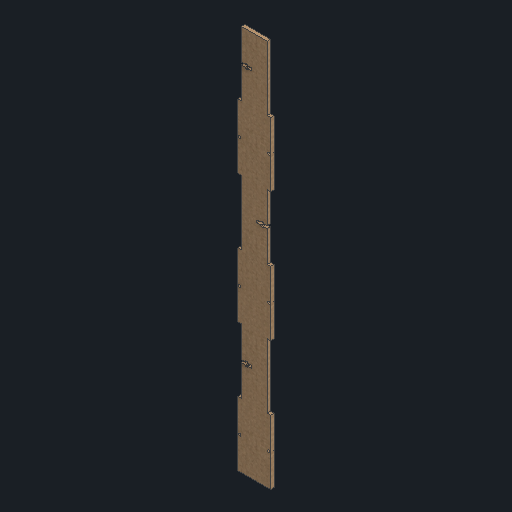
# Autodesk Inventor part: Cableduct_Cover
Saved by Autodesk Inventor 2024.1 (Build 281209000, 209)
## iProperties
Created: 2023-08-04
Part Number: Cableduct_Cover
Material: MDF Medium Density Fiberboard
Document SubType Name: Modeling
Designer: jaege
Density: 0.8 g/cm^3
Appearance: Cardboard - Corrugated
Author: jaege
Autodesk Inventor part; units mm, degrees
ref_plane "YZ Plane" through (0, 0, 0) normal (1, 0, 0) x (0, 1, 0)
ref_plane "XZ Plane" through (0, 0, 0) normal (0, 1, 0) x (-1, 0, 0)
ref_plane "XY Plane" through (0, 0, 0) normal (0, 0, 1) x (1, 0, 0)
sketch "Sketch1" plane through (0, 0, 0) normal (0, 0, 1) x (1, 0, 0)
  line L0 (75.5009, -337.6029) -> (75.5009, -262.6029) projected
  line L1 (71.5009, -262.6029) -> (75.5009, -262.6029) projected
  line L2 (71.5009, -337.6029) -> (71.5009, -262.6029) projected
  line L3 (71.5009, -337.6029) -> (75.5009, -337.6029) projected
  line L4 (75.5009, -187.6029) -> (75.5009, -112.6029) projected
  line L5 (71.5009, -112.6029) -> (75.5009, -112.6029) projected
  line L6 (71.5009, -187.6029) -> (71.5009, -112.6029) projected
  line L7 (71.5009, -187.6029) -> (75.5009, -187.6029) projected
  line L8 (75.5009, -37.6029) -> (75.5009, 37.3971) projected
  line L9 (71.5009, 37.3971) -> (75.5009, 37.3971) projected
  line L10 (71.5009, -37.6029) -> (71.5009, 37.3971) projected
  line L11 (71.5009, -37.6029) -> (75.5009, -37.6029) projected
  line L12 (75.5009, 37.3971) -> (105.5009, 37.3971)
  line L13 (105.5009, 37.3971) -> (105.5009, -412.6029)
  line L14 (105.5009, -412.6029) -> (75.5009, -412.6029)
  line L15 (75.5009, -412.6029) -> (75.5009, 37.3971)
  line L16 (71.5009, -412.6029) -> (279.5009, -412.6029) construction
  line L17 (90.5009, -412.6029) -> (90.5009, 37.3971) construction
  line L18 (105.5009, -337.6029) -> (105.5009, -262.6029)
  line L19 (109.5009, -262.6029) -> (105.5009, -262.6029)
  line L20 (109.5009, -337.6029) -> (109.5009, -262.6029)
  line L21 (109.5009, -337.6029) -> (105.5009, -337.6029)
  line L22 (105.5009, -187.6029) -> (105.5009, -112.6029)
  line L23 (109.5009, -112.6029) -> (105.5009, -112.6029)
  line L24 (109.5009, -187.6029) -> (109.5009, -112.6029)
  line L25 (109.5009, -187.6029) -> (105.5009, -187.6029)
  line L26 (105.5009, -37.6029) -> (105.5009, 37.3971)
  line L27 (109.5009, 37.3971) -> (105.5009, 37.3971)
  line L28 (109.5009, -37.6029) -> (109.5009, 37.3971)
  line L29 (109.5009, -37.6029) -> (105.5009, -37.6029)
  line L30 (71.5009, -37.6029) -> (71.5009, -112.6029)
  line L31 (71.5009, -187.6029) -> (71.5009, -262.6029)
  line L32 (71.5009, -337.6029) -> (71.5009, -412.6029)
  line L33 (75.5009, -412.6029) -> (71.5009, -412.6029)
  line L34 (109.5009, -337.6029) -> (109.5009, -412.6029)
  line L35 (109.5009, -412.6029) -> (105.5009, -412.6029)
  line L36 (109.5009, -262.6029) -> (109.5009, -187.6029)
  line L37 (109.5009, -112.6029) -> (109.5009, -37.6029)
  line L38 (71.5009, -37.6029) -> (75.5009, -112.6029) construction
  circle A0 centre (73.5009, -75.1029) radius 1.5
  circle A1 centre (73.5009, -225.1029) radius 1.5
  circle A2 centre (73.5009, -375.1029) radius 1.5
  circle A3 centre (107.5009, -75.1029) radius 1.5
  circle A4 centre (107.5009, -225.1029) radius 1.5
  circle A5 centre (107.5009, -375.1029) radius 1.5
  line L39 (75.5009, -1.6029) -> (87.5009, -1.6029)
  line L40 (87.5009, -1.6029) -> (87.5009, 1.3971)
  line L41 (87.5009, 1.3971) -> (75.5009, 1.3971)
  line L42 (75.5009, 1.3971) -> (75.5009, -1.6029)
  line L43 (82.7009, 2.5971) -> (80.3009, 2.5971)
  line L44 (80.3009, 2.5971) -> (80.3009, -2.8029)
  line L45 (80.3009, -2.8029) -> (82.7009, -2.8029)
  line L46 (82.7009, -2.8029) -> (82.7009, 2.5971)
  line L47 (93.5009, -151.6029) -> (105.5009, -151.6029)
  line L48 (105.5009, -151.6029) -> (105.5009, -148.6029)
  line L49 (105.5009, -148.6029) -> (93.5009, -148.6029)
  line L50 (93.5009, -148.6029) -> (93.5009, -151.6029)
  line L51 (100.7009, -147.4029) -> (98.3009, -147.4029)
  line L52 (98.3009, -147.4029) -> (98.3009, -152.8029)
  line L53 (98.3009, -152.8029) -> (100.7009, -152.8029)
  line L54 (100.7009, -152.8029) -> (100.7009, -147.4029)
  line L55 (75.5009, -301.6029) -> (87.5009, -301.6029)
  line L56 (87.5009, -301.6029) -> (87.5009, -298.6029)
  line L57 (87.5009, -298.6029) -> (75.5009, -298.6029)
  line L58 (75.5009, -298.6029) -> (75.5009, -301.6029)
  line L59 (82.7009, -297.4029) -> (80.3009, -297.4029)
  line L60 (80.3009, -297.4029) -> (80.3009, -302.8029)
  line L61 (80.3009, -302.8029) -> (82.7009, -302.8029)
  line L62 (82.7009, -302.8029) -> (82.7009, -297.4029)
  point P0 (87.5009, -0.1029)
  point P1 (71.5009, -0.1029)
  point P2 (82.7009, -0.1029)
  point P3 (81.5009, 2.5971)
  point P4 (81.5009, -1.6029)
  point P5 (105.5009, -150.1029)
  point P6 (100.7009, -150.1029)
  point P7 (99.5009, -147.4029)
  point P8 (99.5009, -151.6029)
  point P9 (87.5009, -300.1029)
  point P10 (82.7009, -300.1029)
  point P11 (81.5009, -297.4029)
  point P12 (81.5009, -301.6029)
  point P13 (109.5009, -150.1029)
  point P14 (71.5009, -300.1029)
  point P15 (80.3009, 1.3971)
  point P16 (82.7009, 1.3971)
  point P17 (82.7009, -1.6029)
  point P18 (80.3009, -1.6029)
  point P19 (80.3009, -298.6029)
  point P20 (82.7009, -298.6029)
  point P21 (82.7009, -301.6029)
  point P22 (80.3009, -301.6029)
  point P23 (100.7009, -151.6029)
  point P24 (98.3009, -151.6029)
  point P25 (98.3009, -148.6029)
  point P26 (100.7009, -148.6029)
  dimension "d3" = 30
  dimension "d4" = 3
  dimension "d7" = 150
  dimension "d10" = 34
  dimension "d13" = 3
  dimension "d14" = 12
  dimension "d15" = 5.4
  dimension "d16" = 2.4
  dimension "d17" = 3
  dimension "d18" = 12
  dimension "d19" = 5.4
  dimension "d20" = 2.4
  dimension "d21" = 3
  dimension "d22" = 12
  dimension "d23" = 5.4
  dimension "d24" = 2.4
  constraints: 100 end point, 18 equal length, 18 midpoint, 11 symmetric about line, 10 perpendicular, 8 horizontal, 7 horizontal alignment, 6 centre point, 5 vertical alignment, 3 point on line, 2 vertical, 10 other
  measures "d3" distance of L13.end L14.end
  measures "d4" diameter of A0
  measures "d7" distance of A0.centre A1.centre
  measures "d10" distance of A0.centre A3.centre
  measures "d13" distance of L39.end L40.end
  measures "d14" distance of L40.end L41.end
  measures "d15" distance of L45.end L43.start
  measures "d16" distance of L43.start L43.end
  measures "d17" distance of L47.end L49.start
  measures "d18" distance of L49.start L49.end
  measures "d19" distance of L53.end L54.end
  measures "d20" distance of L54.end L52.start
  measures "d21" distance of L55.end L57.start
  measures "d22" distance of L57.start L57.end
  measures "d23" distance of L61.end L62.end
  measures "d24" distance of L62.end L60.start
extrude "Extrusion1" add sketch "Sketch1" along normal blind 4 contours L15 L33 L32 L3 | L0 L55 L60 L61 L62 L56 L57 L59 L15 L4 L8 L39 L44 L45 L46 L40 L41 L43 L12 L13 L49 L54 L51 L52 L50 L47 L53 L14 | L31 L7 L15 L1 | L13 L21 L34 L35 | L30 L11 L15 L5 | L13 L25 L36 L19 | L23 L13 L29 L37
body "Solid1"
